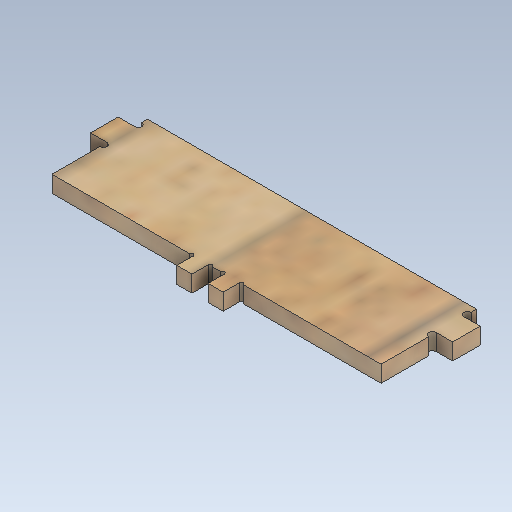
# Autodesk Inventor part: Support A Cross Dual2
Saved by Autodesk Inventor 2020 (Build 240168000, 168)
## iProperties
Created: 2020-03-07
Part Number: Support A Cross Dual2
Material: Wood (Maple)
Document SubType Name: Modeling
Designer: Daniel Wikman
Density: 0.67 g/cm^3
Appearance: Natural Maple - Glossy Dark Tint
Author: Daniel Wikman
Autodesk Inventor part; units mm, degrees
ref_plane "YZ Plane" through (0, 0, 0) normal (1, 0, 0) x (0, 1, 0)
ref_plane "XZ Plane" through (0, 0, 0) normal (0, 1, 0) x (-1, 0, 0)
ref_plane "XY Plane" through (0, 0, 0) normal (0, 0, 1) x (1, 0, 0)
sketch "Sketch1" plane through (0, 0, 0) normal (0, 1, 0) x (-1, 0, 0)
  line L0 (54.4292, -43.2642) -> (54.4292, -41.2642)
  arc A0 (54.4292, -38.5976) -> (54.4292, -41.2642) centre (54.4292, -39.9309) ccw
  arc A1 (54.4292, -25.9309) -> (54.4292, -28.5976) centre (54.4292, -27.2642) ccw
  line L1 (54.4292, -25.9309) -> (54.4292, -8.5976)
  line L2 (54.4292, -28.5976) -> (60.4292, -28.5976)
  line L3 (54.4292, -38.5976) -> (60.4292, -38.5976)
  line L4 (60.4292, -38.5976) -> (60.4292, -28.5976)
  line L5 (54.4292, -43.2642) -> (-65.0708, -43.2642)
  line L6 (-65.0708, -43.2642) -> (-65.0708, -41.2642)
  arc A2 (-65.0708, -41.2642) -> (-65.0708, -38.5976) centre (-65.0708, -39.9309) ccw
  arc A3 (-65.0708, -28.5976) -> (-65.0708, -25.9309) centre (-65.0708, -27.2642) ccw
  line L7 (-65.0708, -25.9309) -> (-65.0708, -8.5976)
  line L8 (-65.0708, -28.5976) -> (-71.0708, -28.5976)
  line L9 (-65.0708, -38.5976) -> (-71.0708, -38.5976)
  line L10 (-71.0708, -38.5976) -> (-71.0708, -28.5976)
  line L11 (-21.0708, -8.5976) -> (-65.0708, -8.5976)
  line L12 (54.4292, -8.5976) -> (10.4292, -8.5976)
  line L13 (-19.7375, -2.5976) -> (9.0959, -2.5976)
  line L14 (-19.7375, -8.5976) -> (-19.7375, -2.5976)
  line L15 (9.0959, -8.5976) -> (9.0959, -2.5976)
  line L16 (-21.0708, -8.5976) -> (-19.7375, -8.5976)
  line L17 (10.4292, -8.5976) -> (9.0959, -8.5976)
  point P0 (0, 0)
  dimension "d1" = 2
  dimension "d2" = 2.6667
  dimension "d5" = 2.6667
  dimension "d6" = 17.3333
  dimension "d9" = 6
  dimension "d10" = 119.5
  dimension "d11" = 10
  dimension "d18" = 44
  dimension "d19" = 44
  dimension "d21" = 20
  dimension "d23" = 6
  constraints: 36 end point, 8 horizontal, 8 point on circle, 4 centre point, 4 vertical, 1 perpendicular
  measures "d1" distance of L0.start L0.end
  measures "d2" diameter of A0
  measures "d5" diameter of A1
  measures "d6" distance of L1.start L1.end
  measures "d9" distance of L2.start L2.end
  measures "d10" distance of L0.start L5.end
  measures "d11" distance of L3.end L2.end
  measures "d18" distance of L1.end L12.end
  measures "d19" distance of L11.start L7.end
  measures "d21" distance between parallel lines of L2 L12
  measures "d23" distance between parallel lines of L12 L13
extrude "Extrusion1" add sketch "Sketch1" along normal blind 6
sketch "Sketch2" plane through (0, 6, 0) normal (0, 1, 0) x (1, 0, 0)
  line L0 (2.4041, 2.5976) -> (2.4041, 8.5976)
  line L1 (-3.0959, 8.5976) -> (-3.0959, 2.5976)
  line L2 (-9.0959, 8.5976) -> (-9.0959, 2.5976) projected
  line L3 (13.7375, 8.5976) -> (13.7375, 2.5976)
  line L4 (8.2375, 2.5976) -> (8.2375, 8.5976)
  line L5 (19.7375, 2.5976) -> (19.7375, 8.5976) projected
  line L6 (-9.0959, 8.5976) -> (-4.4292, 8.5976)
  line L7 (-3.0959, 8.5976) -> (-3.0959, 2.5976)
  line L8 (-3.0959, 2.5976) -> (-9.0959, 2.5976)
  line L9 (-9.0959, 2.5976) -> (-9.0959, 8.5976)
  line L10 (3.7375, 8.5976) -> (6.9041, 8.5976)
  line L11 (8.2375, 8.5976) -> (8.2375, 2.5976)
  line L12 (8.2375, 2.5976) -> (2.4041, 2.5976)
  line L13 (2.4041, 2.5976) -> (2.4041, 8.5976)
  line L14 (15.0708, 8.5976) -> (19.7375, 8.5976)
  line L15 (19.7375, 8.5976) -> (19.7375, 2.5976)
  line L16 (19.7375, 2.5976) -> (13.7375, 2.5976)
  line L17 (13.7375, 2.5976) -> (13.7375, 8.5976)
  arc A0 (3.7375, 8.5976) -> (2.4041, 8.5976) centre (3.0708, 8.5976) ccw
  arc A1 (8.2375, 8.5976) -> (6.9041, 8.5976) centre (7.5708, 8.5976) ccw
  arc A2 (-3.0959, 8.5976) -> (-4.4292, 8.5976) centre (-3.7625, 8.5976) ccw
  arc A3 (15.0708, 8.5976) -> (13.7375, 8.5976) centre (14.4041, 8.5976) ccw
  point P0 (0, 0)
  dimension "d26" = 6
  dimension "d28" = 6
  dimension "d29" = 6
  dimension "d37" = 1.3333
  dimension "d38" = 1.3333
  dimension "d39" = 1.3333
  dimension "d40" = 1.3333
  constraints: 32 end point, 8 parallel, 8 point on circle, 4 centre point, 4 point on line, 3 horizontal, 3 perpendicular
  measures "d26" distance of L1.start L1.end
  measures "d28" distance between parallel lines of L2 L1
  measures "d29" distance between parallel lines of L5 L3
  measures "d37" diameter of A0
  measures "d38" diameter of A1
  measures "d39" diameter of A2
  measures "d40" diameter of A3
extrude "Extrusion2" cut sketch "Sketch2" against normal through all
body "Solid1"
